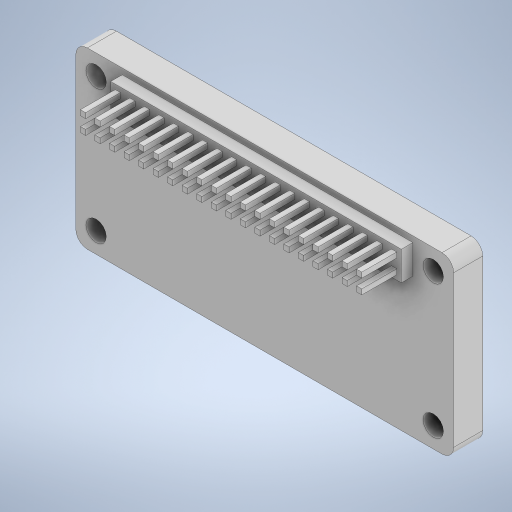
# Autodesk Inventor part: OrangePi
Saved by Autodesk Inventor 2024 (Build 280153000, 153)
## iProperties
Created: 2024-03-12
Part Number: OrangePi
Material: Générique
Document SubType Name: Modeling
Designer: phaly
Density: 1 g/cm^3
Appearance: Par défaut
Author: phaly
Autodesk Inventor part; units mm, degrees
ref_plane "YZ Plane" through (0, 0, 0) normal (1, 0, 0) x (0, 1, 0)
ref_plane "XZ Plane" through (0, 0, 0) normal (0, 1, 0) x (-1, 0, 0)
ref_plane "XY Plane" through (0, 0, 0) normal (0, 0, 1) x (1, 0, 0)
sketch "Esquisse1" plane through (0, 0, 0) normal (0, 0, 1) x (1, 0, 0)
  line L0 (0, 30) -> (65, 30)
  line L1 (65, 30) -> (65, 0)
  line L2 (65, 0) -> (0, 0)
  line L3 (0, 0) -> (0, 30)
  line L4 (-13, 0) -> (78, 0) projected
  line L5 (0, -6) -> (0, 36) projected
  point P0 (0, 0)
  dimension "d0" = 65
  dimension "d1" = 30
  constraints: 8 end point, 2 collinear, 2 parallel, 1 horizontal, 1 perpendicular
  measures "d0" distance of L0.start L0.end
  measures "d1" distance between parallel lines of L2 L0
extrude "Extrusion1" add sketch "Esquisse1" along normal mid plane 5
sketch "Esquisse2" plane through (0, 0, 2.5) normal (0, 0, 1) x (1, 0, 0)
  line L0 (0, 30) -> (0, 0) projected
  line L1 (0, 0) -> (65, 0) projected
  line L2 (65, 30) -> (0, 30) projected
  point P0 (3.5, 26.5)
  point P1 (61.5, 26.5)
  point P2 (61.5, 3.5)
  point P3 (3.5, 3.5)
  dimension "d4" = 58
  dimension "d5" = 23
  dimension "d6" = 23
  dimension "d7" = 58
  dimension "d8" = 3.5
  dimension "d9" = 3.5
  dimension "d10" = 3.5
  dimension "d11" = 3.5
  measures "d4" distance of point (61.5, 26.5) point (3.5, 26.5)
  measures "d5" distance of point (3.5, 3.5) point (3.5, 26.5)
  measures "d6" distance of point (61.5, 3.5) point (61.5, 26.5)
  measures "d7" distance of point (3.5, 3.5) point (61.5, 3.5)
  measures "d8" distance from line of L0 point (3.5, 26.5)
  measures "d9" distance from line of L0 point (3.5, 3.5)
  measures "d10" distance from line of L1 point (3.5, 3.5)
  measures "d11" distance from line of L2 point (61.5, 26.5)
hole "Perçage1" at (3.5, 26.5, 2.5) at (61.5, 26.5, 2.5) at (61.5, 3.5, 2.5) at (3.5, 3.5, 2.5) direction (0, 0, -1) diameter 3.5 end through all
sketch "Esquisse3" plane through (0, 0, 2.5) normal (0, 0, 1) x (1, 0, 0)
  line L0 (8, 29) -> (10.5, 29)
  line L1 (10.5, 29) -> (10.5, 26.5)
  line L2 (10.5, 26.5) -> (8, 26.5)
  line L3 (8, 26.5) -> (8, 29)
  line L4 (8, 26.5) -> (10.5, 26.5)
  line L5 (10.5, 26.5) -> (10.5, 24)
  line L6 (10.5, 24) -> (8, 24)
  line L7 (8, 24) -> (8, 26.5)
  line L8 (65, 30) -> (0, 30) projected
  line L9 (0, 30) -> (0, 0) projected
  line L10 (10.5, 29) -> (13, 29)
  line L11 (10.5, 26.5) -> (10.5, 29)
  line L12 (13, 29) -> (13, 26.5)
  line L13 (13, 26.5) -> (10.5, 26.5)
  line L14 (13, 26.5) -> (13, 24)
  line L15 (13, 24) -> (10.5, 24)
  line L16 (10.5, 24) -> (10.5, 26.5)
  line L17 (13, 29) -> (15.5, 29)
  line L18 (13, 26.5) -> (13, 29)
  line L19 (15.5, 29) -> (15.5, 26.5)
  line L20 (15.5, 26.5) -> (13, 26.5)
  line L21 (15.5, 26.5) -> (15.5, 24)
  line L22 (15.5, 24) -> (13, 24)
  line L23 (13, 24) -> (13, 26.5)
  line L24 (15.5, 29) -> (18, 29)
  line L25 (15.5, 26.5) -> (15.5, 29)
  line L26 (18, 29) -> (18, 26.5)
  line L27 (18, 26.5) -> (15.5, 26.5)
  line L28 (18, 26.5) -> (18, 24)
  line L29 (18, 24) -> (15.5, 24)
  line L30 (15.5, 24) -> (15.5, 26.5)
  line L31 (18, 29) -> (20.5, 29)
  line L32 (18, 26.5) -> (18, 29)
  line L33 (20.5, 29) -> (20.5, 26.5)
  line L34 (20.5, 26.5) -> (18, 26.5)
  line L35 (20.5, 26.5) -> (20.5, 24)
  line L36 (20.5, 24) -> (18, 24)
  line L37 (18, 24) -> (18, 26.5)
  line L38 (20.5, 29) -> (23, 29)
  line L39 (20.5, 26.5) -> (20.5, 29)
  line L40 (23, 29) -> (23, 26.5)
  line L41 (23, 26.5) -> (20.5, 26.5)
  line L42 (23, 26.5) -> (23, 24)
  line L43 (23, 24) -> (20.5, 24)
  line L44 (20.5, 24) -> (20.5, 26.5)
  line L45 (23, 29) -> (25.5, 29)
  line L46 (23, 26.5) -> (23, 29)
  line L47 (25.5, 29) -> (25.5, 26.5)
  line L48 (25.5, 26.5) -> (23, 26.5)
  line L49 (25.5, 26.5) -> (25.5, 24)
  line L50 (25.5, 24) -> (23, 24)
  line L51 (23, 24) -> (23, 26.5)
  line L52 (25.5, 29) -> (28, 29)
  line L53 (25.5, 26.5) -> (25.5, 29)
  line L54 (28, 29) -> (28, 26.5)
  line L55 (28, 26.5) -> (25.5, 26.5)
  line L56 (28, 26.5) -> (28, 24)
  line L57 (28, 24) -> (25.5, 24)
  line L58 (25.5, 24) -> (25.5, 26.5)
  line L59 (28, 29) -> (30.5, 29)
  line L60 (28, 26.5) -> (28, 29)
  line L61 (30.5, 29) -> (30.5, 26.5)
  line L62 (30.5, 26.5) -> (28, 26.5)
  line L63 (30.5, 26.5) -> (30.5, 24)
  line L64 (30.5, 24) -> (28, 24)
  line L65 (28, 24) -> (28, 26.5)
  line L66 (30.5, 29) -> (33, 29)
  line L67 (30.5, 26.5) -> (30.5, 29)
  line L68 (33, 29) -> (33, 26.5)
  line L69 (33, 26.5) -> (30.5, 26.5)
  line L70 (33, 26.5) -> (33, 24)
  line L71 (33, 24) -> (30.5, 24)
  line L72 (30.5, 24) -> (30.5, 26.5)
  line L73 (33, 29) -> (35.5, 29)
  line L74 (33, 26.5) -> (33, 29)
  line L75 (35.5, 29) -> (35.5, 26.5)
  line L76 (35.5, 26.5) -> (33, 26.5)
  line L77 (35.5, 26.5) -> (35.5, 24)
  line L78 (35.5, 24) -> (33, 24)
  line L79 (33, 24) -> (33, 26.5)
  line L80 (35.5, 29) -> (38, 29)
  line L81 (35.5, 26.5) -> (35.5, 29)
  line L82 (38, 29) -> (38, 26.5)
  line L83 (38, 26.5) -> (35.5, 26.5)
  line L84 (38, 26.5) -> (38, 24)
  line L85 (38, 24) -> (35.5, 24)
  line L86 (35.5, 24) -> (35.5, 26.5)
  line L87 (38, 29) -> (40.5, 29)
  line L88 (38, 26.5) -> (38, 29)
  line L89 (40.5, 29) -> (40.5, 26.5)
  line L90 (40.5, 26.5) -> (38, 26.5)
  line L91 (40.5, 26.5) -> (40.5, 24)
  line L92 (40.5, 24) -> (38, 24)
  line L93 (38, 24) -> (38, 26.5)
  line L94 (40.5, 29) -> (43, 29)
  line L95 (40.5, 26.5) -> (40.5, 29)
  line L96 (43, 29) -> (43, 26.5)
  line L97 (43, 26.5) -> (40.5, 26.5)
  line L98 (43, 26.5) -> (43, 24)
  line L99 (43, 24) -> (40.5, 24)
  line L100 (40.5, 24) -> (40.5, 26.5)
  line L101 (43, 29) -> (45.5, 29)
  line L102 (43, 26.5) -> (43, 29)
  line L103 (45.5, 29) -> (45.5, 26.5)
  line L104 (45.5, 26.5) -> (43, 26.5)
  line L105 (45.5, 26.5) -> (45.5, 24)
  line L106 (45.5, 24) -> (43, 24)
  line L107 (43, 24) -> (43, 26.5)
  line L108 (45.5, 29) -> (48, 29)
  line L109 (45.5, 26.5) -> (45.5, 29)
  line L110 (48, 29) -> (48, 26.5)
  line L111 (48, 26.5) -> (45.5, 26.5)
  line L112 (48, 26.5) -> (48, 24)
  line L113 (48, 24) -> (45.5, 24)
  line L114 (45.5, 24) -> (45.5, 26.5)
  line L115 (48, 29) -> (50.5, 29)
  line L116 (48, 26.5) -> (48, 29)
  line L117 (50.5, 29) -> (50.5, 26.5)
  line L118 (50.5, 26.5) -> (48, 26.5)
  line L119 (50.5, 26.5) -> (50.5, 24)
  line L120 (50.5, 24) -> (48, 24)
  line L121 (48, 24) -> (48, 26.5)
  line L122 (50.5, 29) -> (53, 29)
  line L123 (50.5, 26.5) -> (50.5, 29)
  line L124 (53, 29) -> (53, 26.5)
  line L125 (53, 26.5) -> (50.5, 26.5)
  line L126 (53, 26.5) -> (53, 24)
  line L127 (53, 24) -> (50.5, 24)
  line L128 (50.5, 24) -> (50.5, 26.5)
  line L129 (53, 29) -> (55.5, 29)
  line L130 (53, 26.5) -> (53, 29)
  line L131 (55.5, 29) -> (55.5, 26.5)
  line L132 (55.5, 26.5) -> (53, 26.5)
  line L133 (55.5, 26.5) -> (55.5, 24)
  line L134 (55.5, 24) -> (53, 24)
  line L135 (53, 24) -> (53, 26.5)
  line L136 (55.5, 29) -> (58, 29)
  line L137 (55.5, 26.5) -> (55.5, 29)
  line L138 (58, 29) -> (58, 26.5)
  line L139 (58, 26.5) -> (55.5, 26.5)
  line L140 (58, 26.5) -> (58, 24)
  line L141 (58, 24) -> (55.5, 24)
  line L142 (55.5, 24) -> (55.5, 26.5)
  dimension "d19" = 2.5
  dimension "d22" = 1
  dimension "d23" = 8
  dimension "d26" = 2.5
  dimension "d31" = 5
  dimension "d32" = 2.5
  constraints: 282 end point, 40 point on line, 4 parallel, 3 horizontal, 2 perpendicular, 1 collinear, 285 other
  measures "d19" distance of L0.start L0.end
  measures "d22" distance between parallel lines of L8 L0
  measures "d23" distance between parallel lines of L9 L3
  measures "d26" distance of L0.start L10.start
  measures "d31" distance between parallel lines of L6 L0
  measures "d32" distance between parallel lines of L6 L2
extrude "Extrusion2" add sketch "Esquisse3" along normal blind 2
sketch "Esquisse4" plane through (0, 0, 4.5) normal (0, 0, 1) x (1, 0, 0)
  line L0 (8.8, 28.2) -> (9.7, 28.2)
  line L1 (9.7, 28.2) -> (9.7, 27.3)
  line L2 (9.7, 27.3) -> (8.8, 27.3)
  line L3 (8.8, 27.3) -> (8.8, 28.2)
  line L4 (8.8, 25.7) -> (9.7, 25.7)
  line L5 (9.7, 25.7) -> (9.7, 24.8)
  line L6 (9.7, 24.8) -> (8.8, 24.8)
  line L7 (8.8, 24.8) -> (8.8, 25.7)
  line L8 (8, 24) -> (58, 24) projected
  line L9 (8, 29) -> (8, 24) projected
  line L10 (58, 29) -> (8, 29) projected
  line L11 (12.2, 27.3) -> (11.3, 27.3)
  line L12 (12.2, 28.2) -> (12.2, 27.3)
  line L13 (11.3, 28.2) -> (12.2, 28.2)
  line L14 (11.3, 27.3) -> (11.3, 28.2)
  line L15 (11.3, 25.7) -> (12.2, 25.7)
  line L16 (12.2, 25.7) -> (12.2, 24.8)
  line L17 (12.2, 24.8) -> (11.3, 24.8)
  line L18 (11.3, 24.8) -> (11.3, 25.7)
  line L19 (14.7, 27.3) -> (13.8, 27.3)
  line L20 (14.7, 28.2) -> (14.7, 27.3)
  line L21 (13.8, 28.2) -> (14.7, 28.2)
  line L22 (13.8, 27.3) -> (13.8, 28.2)
  line L23 (13.8, 25.7) -> (14.7, 25.7)
  line L24 (14.7, 25.7) -> (14.7, 24.8)
  line L25 (14.7, 24.8) -> (13.8, 24.8)
  line L26 (13.8, 24.8) -> (13.8, 25.7)
  line L27 (17.2, 27.3) -> (16.3, 27.3)
  line L28 (17.2, 28.2) -> (17.2, 27.3)
  line L29 (16.3, 28.2) -> (17.2, 28.2)
  line L30 (16.3, 27.3) -> (16.3, 28.2)
  line L31 (16.3, 25.7) -> (17.2, 25.7)
  line L32 (17.2, 25.7) -> (17.2, 24.8)
  line L33 (17.2, 24.8) -> (16.3, 24.8)
  line L34 (16.3, 24.8) -> (16.3, 25.7)
  line L35 (19.7, 27.3) -> (18.8, 27.3)
  line L36 (19.7, 28.2) -> (19.7, 27.3)
  line L37 (18.8, 28.2) -> (19.7, 28.2)
  line L38 (18.8, 27.3) -> (18.8, 28.2)
  line L39 (18.8, 25.7) -> (19.7, 25.7)
  line L40 (19.7, 25.7) -> (19.7, 24.8)
  line L41 (19.7, 24.8) -> (18.8, 24.8)
  line L42 (18.8, 24.8) -> (18.8, 25.7)
  line L43 (22.2, 27.3) -> (21.3, 27.3)
  line L44 (22.2, 28.2) -> (22.2, 27.3)
  line L45 (21.3, 28.2) -> (22.2, 28.2)
  line L46 (21.3, 27.3) -> (21.3, 28.2)
  line L47 (21.3, 25.7) -> (22.2, 25.7)
  line L48 (22.2, 25.7) -> (22.2, 24.8)
  line L49 (22.2, 24.8) -> (21.3, 24.8)
  line L50 (21.3, 24.8) -> (21.3, 25.7)
  line L51 (24.7, 27.3) -> (23.8, 27.3)
  line L52 (24.7, 28.2) -> (24.7, 27.3)
  line L53 (23.8, 28.2) -> (24.7, 28.2)
  line L54 (23.8, 27.3) -> (23.8, 28.2)
  line L55 (23.8, 25.7) -> (24.7, 25.7)
  line L56 (24.7, 25.7) -> (24.7, 24.8)
  line L57 (24.7, 24.8) -> (23.8, 24.8)
  line L58 (23.8, 24.8) -> (23.8, 25.7)
  line L59 (27.2, 27.3) -> (26.3, 27.3)
  line L60 (27.2, 28.2) -> (27.2, 27.3)
  line L61 (26.3, 28.2) -> (27.2, 28.2)
  line L62 (26.3, 27.3) -> (26.3, 28.2)
  line L63 (26.3, 25.7) -> (27.2, 25.7)
  line L64 (27.2, 25.7) -> (27.2, 24.8)
  line L65 (27.2, 24.8) -> (26.3, 24.8)
  line L66 (26.3, 24.8) -> (26.3, 25.7)
  line L67 (29.7, 27.3) -> (28.8, 27.3)
  line L68 (29.7, 28.2) -> (29.7, 27.3)
  line L69 (28.8, 28.2) -> (29.7, 28.2)
  line L70 (28.8, 27.3) -> (28.8, 28.2)
  line L71 (28.8, 25.7) -> (29.7, 25.7)
  line L72 (29.7, 25.7) -> (29.7, 24.8)
  line L73 (29.7, 24.8) -> (28.8, 24.8)
  line L74 (28.8, 24.8) -> (28.8, 25.7)
  line L75 (32.2, 27.3) -> (31.3, 27.3)
  line L76 (32.2, 28.2) -> (32.2, 27.3)
  line L77 (31.3, 28.2) -> (32.2, 28.2)
  line L78 (31.3, 27.3) -> (31.3, 28.2)
  line L79 (31.3, 25.7) -> (32.2, 25.7)
  line L80 (32.2, 25.7) -> (32.2, 24.8)
  line L81 (32.2, 24.8) -> (31.3, 24.8)
  line L82 (31.3, 24.8) -> (31.3, 25.7)
  line L83 (34.7, 27.3) -> (33.8, 27.3)
  line L84 (34.7, 28.2) -> (34.7, 27.3)
  line L85 (33.8, 28.2) -> (34.7, 28.2)
  line L86 (33.8, 27.3) -> (33.8, 28.2)
  line L87 (33.8, 25.7) -> (34.7, 25.7)
  line L88 (34.7, 25.7) -> (34.7, 24.8)
  line L89 (34.7, 24.8) -> (33.8, 24.8)
  line L90 (33.8, 24.8) -> (33.8, 25.7)
  line L91 (37.2, 27.3) -> (36.3, 27.3)
  line L92 (37.2, 28.2) -> (37.2, 27.3)
  line L93 (36.3, 28.2) -> (37.2, 28.2)
  line L94 (36.3, 27.3) -> (36.3, 28.2)
  line L95 (36.3, 25.7) -> (37.2, 25.7)
  line L96 (37.2, 25.7) -> (37.2, 24.8)
  line L97 (37.2, 24.8) -> (36.3, 24.8)
  line L98 (36.3, 24.8) -> (36.3, 25.7)
  line L99 (39.7, 27.3) -> (38.8, 27.3)
  line L100 (39.7, 28.2) -> (39.7, 27.3)
  line L101 (38.8, 28.2) -> (39.7, 28.2)
  line L102 (38.8, 27.3) -> (38.8, 28.2)
  line L103 (38.8, 25.7) -> (39.7, 25.7)
  line L104 (39.7, 25.7) -> (39.7, 24.8)
  line L105 (39.7, 24.8) -> (38.8, 24.8)
  line L106 (38.8, 24.8) -> (38.8, 25.7)
  line L107 (42.2, 27.3) -> (41.3, 27.3)
  line L108 (42.2, 28.2) -> (42.2, 27.3)
  line L109 (41.3, 28.2) -> (42.2, 28.2)
  line L110 (41.3, 27.3) -> (41.3, 28.2)
  line L111 (41.3, 25.7) -> (42.2, 25.7)
  line L112 (42.2, 25.7) -> (42.2, 24.8)
  line L113 (42.2, 24.8) -> (41.3, 24.8)
  line L114 (41.3, 24.8) -> (41.3, 25.7)
  line L115 (44.7, 27.3) -> (43.8, 27.3)
  line L116 (44.7, 28.2) -> (44.7, 27.3)
  line L117 (43.8, 28.2) -> (44.7, 28.2)
  line L118 (43.8, 27.3) -> (43.8, 28.2)
  line L119 (43.8, 25.7) -> (44.7, 25.7)
  line L120 (44.7, 25.7) -> (44.7, 24.8)
  line L121 (44.7, 24.8) -> (43.8, 24.8)
  line L122 (43.8, 24.8) -> (43.8, 25.7)
  line L123 (47.2, 27.3) -> (46.3, 27.3)
  line L124 (47.2, 28.2) -> (47.2, 27.3)
  line L125 (46.3, 28.2) -> (47.2, 28.2)
  line L126 (46.3, 27.3) -> (46.3, 28.2)
  line L127 (46.3, 25.7) -> (47.2, 25.7)
  line L128 (47.2, 25.7) -> (47.2, 24.8)
  line L129 (47.2, 24.8) -> (46.3, 24.8)
  line L130 (46.3, 24.8) -> (46.3, 25.7)
  line L131 (49.7, 27.3) -> (48.8, 27.3)
  line L132 (49.7, 28.2) -> (49.7, 27.3)
  line L133 (48.8, 28.2) -> (49.7, 28.2)
  line L134 (48.8, 27.3) -> (48.8, 28.2)
  line L135 (48.8, 25.7) -> (49.7, 25.7)
  line L136 (49.7, 25.7) -> (49.7, 24.8)
  line L137 (49.7, 24.8) -> (48.8, 24.8)
  line L138 (48.8, 24.8) -> (48.8, 25.7)
  line L139 (52.2, 27.3) -> (51.3, 27.3)
  line L140 (52.2, 28.2) -> (52.2, 27.3)
  line L141 (51.3, 28.2) -> (52.2, 28.2)
  line L142 (51.3, 27.3) -> (51.3, 28.2)
  line L143 (51.3, 25.7) -> (52.2, 25.7)
  line L144 (52.2, 25.7) -> (52.2, 24.8)
  line L145 (52.2, 24.8) -> (51.3, 24.8)
  line L146 (51.3, 24.8) -> (51.3, 25.7)
  line L147 (54.7, 27.3) -> (53.8, 27.3)
  line L148 (54.7, 28.2) -> (54.7, 27.3)
  line L149 (53.8, 28.2) -> (54.7, 28.2)
  line L150 (53.8, 27.3) -> (53.8, 28.2)
  line L151 (53.8, 25.7) -> (54.7, 25.7)
  line L152 (54.7, 25.7) -> (54.7, 24.8)
  line L153 (54.7, 24.8) -> (53.8, 24.8)
  line L154 (53.8, 24.8) -> (53.8, 25.7)
  line L155 (57.2, 27.3) -> (56.3, 27.3)
  line L156 (57.2, 28.2) -> (57.2, 27.3)
  line L157 (56.3, 28.2) -> (57.2, 28.2)
  line L158 (56.3, 27.3) -> (56.3, 28.2)
  line L159 (56.3, 25.7) -> (57.2, 25.7)
  line L160 (57.2, 25.7) -> (57.2, 24.8)
  line L161 (57.2, 24.8) -> (56.3, 24.8)
  line L162 (56.3, 24.8) -> (56.3, 25.7)
  point P0 (0, 0)
  dimension "d35" = 0.9
  dimension "d36" = 0.9
  dimension "d37" = 0.9
  dimension "d38" = 0.9
  dimension "d40" = 0.8
  dimension "d41" = 0.8
  dimension "d42" = 0.8
  dimension "d45" = 2.5
  constraints: 320 end point, 20 point on line, 4 parallel, 3 horizontal, 2 perpendicular, 304 other
  measures "d35" distance of L0.start L0.end
  measures "d36" distance of L4.start L4.end
  measures "d37" distance of L6.end L4.start
  measures "d38" distance of L2.end L0.start
  measures "d40" distance between parallel lines of L8 L6
  measures "d41" distance between parallel lines of L9 L7
  measures "d42" distance between parallel lines of L10 L0
  measures "d45" distance of L1.end L11.start
extrude "Extrusion3" add sketch "Esquisse4" along normal blind 6
fillet "Congé1" radius 2 4 edges at (0, 0, 0) (65, 0, 0) (65, 30, 0) (0, 30, 0)
equation "\"d6\" = d5"
equation "\"d7\" = d4"
equation "\"d9\" = d8"
equation "\"d10\" = d9"
equation "\"d11\" = d8"
equation "\"d19\" = d32"
equation "\"d32\" = 0.5 * d31"
equation "\"d37\" = d36"
equation "\"d38\" = d35"
equation "\"d42\" = d40"
